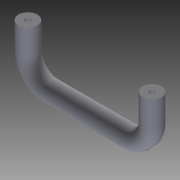
# Autodesk Inventor part: FrameHandle
Saved by Autodesk Inventor 2015 SP1 (Build 190203100, 203)
## iProperties
Created: 2015-03-15
Part Number: FrameHandle
Material: ABS Plastic
Document SubType Name: Modeling
Designer: Jack
Density: 1.06 g/cm^3
Appearance: Cyan
Author: Jack
Autodesk Inventor part; units mm, degrees
ref_plane "YZ Plane" through (0, 0, 0) normal (1, 0, 0) x (0, 1, 0)
ref_plane "XZ Plane" through (0, 0, 0) normal (0, 1, 0) x (-1, 0, 0)
ref_plane "XY Plane" through (0, 0, 0) normal (0, 0, 1) x (1, 0, 0)
sketch "Sketch1" plane through (0, 0, 0) normal (0, 0, 1) x (1, 0, 0)
  circle A0 centre (0, 0) radius 8
  dimension "d0" = 16
  constraints: 1 centre point, 1 coincident
  measures "d0" diameter of A0
sketch "Sketch2" plane through (0, 0, 0) normal (0, 1, 0) x (-1, 0, 0)
  line L0 (0, 0) -> (0, -22)
  line L1 (-20, -42) -> (-85, -42)
  line L2 (-105, -22) -> (-105, 0)
  arc A0 (-20, -42) -> (0, -22) centre (-20, -22) ccw
  arc A1 (-105, -22) -> (-85, -42) centre (-85, -22) ccw
  point P0 (0, -42)
  point P1 (-105, -42)
  dimension "d1" = 105
  dimension "d2" = 42
  dimension "d3" = 20
  constraints: 6 end point, 4 point on circle, 4 point on line, 4 tangent, 2 centre point, 2 perpendicular, 1 equal radius, 1 horizontal alignment, 1 vertical
  measures "d1" distance of point (0, -42) point (-105, -42)
  measures "d2" distance of L0.start point (0, -42)
  measures "d3" radius of A0
sweep "Sweep1" add profiles "Sketch1" path "Sketch2" path curves L0 A0 L1 A1 L2
ref_plane "Work Plane1" through (0, 0, -55) normal (0, 0, 1) x (1, 0, 0)
sketch "Sketch3" plane through (0, 0, -55) normal (0, 0, 1) x (1, 0, 0)
  circle A0 centre (0, 0) radius 3.7
  circle A1 centre (105, 0) radius 8 projected
  circle A2 centre (105, 0) radius 3.7
  dimension "d7" = 7.4
  dimension "d8" = 7.4
  constraints: 2 centre point, 2 coincident
  measures "d7" diameter of A0
  measures "d8" diameter of A2
extrude "Extrusion1" cut sketch "Sketch3" along normal blind 49 contours A0 | A2
sketch "Sketch4" plane through (0, 0, -6) normal (0, 0, -1) x (-1, 0, 0)
  circle A0 centre (0, 0) radius 3.7 projected
  circle A1 centre (-105, 0) radius 3.7 projected
  circle A2 centre (0, 0) radius 2.25
  circle A3 centre (-105, 0) radius 2.25
  dimension "d11" = 4.5
  dimension "d12" = 4.5
  constraints: 2 centre point, 2 coincident
  measures "d11" diameter of A2
  measures "d12" diameter of A3
extrude "Extrusion2" cut sketch "Sketch4" against normal up to surface (6 mm away) contours A2 | A3
body "Solid1"
